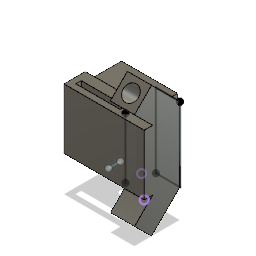
batt basee v1 (Autodesk Fusion 360 design; units mm, degrees)
Autodesk Fusion 360 part; units mm, degrees
sketch "Sketch1" plane through (0, 0, 0) normal (0, 0, 1) x (1, 0, 0)
  line L0 (0, 0) -> (13.5, 0)
  line L1 (13.5, 0) -> (13.5, 13.5)
  line L2 (13.5, 13.5) -> (0, 13.5)
  line L3 (0, 13.5) -> (0, 0)
  line L4 (-3.75, -3.75) -> (17.25, -3.75)
  line L5 (17.25, -3.75) -> (17.25, 17.25)
  line L6 (17.25, 17.25) -> (-3.75, 17.25)
  line L7 (-3.75, 17.25) -> (-3.75, -3.75)
  dimension "d1" = 13.5
  dimension "d2" = 13.5
  dimension "d3" = 3.75
  constraint horizontal L0
  constraint vertical L1
  constraint horizontal L2
  constraint vertical L3
  constraint coincident L0.start L3.end
  measures "d1" distance of L0.start L2.end
  measures "d2" distance of L1.end L2.end
  measures "d43" distance of L0.start
  measures "d47" distance of L0.start
extrude "Extrude1" add sketch "Sketch1" along normal blind 20
sketch "Sketch2" plane through (0, 0, 20) normal (0, 0, 1) x (1, 0, 0)
  line L0 (0, 0) -> (0, 13.5)
  line L1 (0, 13.5) -> (13.5, 13.5)
  line L2 (13.5, 13.5) -> (13.5, 0)
  line L3 (13.5, 0) -> (0, 0)
  line L4 (-3.75, 17.25) -> (-3.75, -3.75)
  line L5 (-3.75, -3.75) -> (17.25, -3.75)
  line L6 (17.25, -3.75) -> (17.25, 17.25)
  line L7 (17.25, 17.25) -> (-3.75, 17.25)
  line L8 (6.75, 6.75) -> (6.75, 21.75)
  line L9 (6.75, 6.75) -> (6.75, -8.25)
  line L10 (6.75, 6.75) -> (17.25, 6.75)
  line L11 (17.25, 6.75) -> (17.25, 21.75)
  line L12 (17.25, 21.75) -> (6.75, 21.75)
  line L13 (6.75, -8.25) -> (17.25, -8.25)
  line L14 (17.25, -8.25) -> (17.25, 6.75)
  line L15 (6.75, 6.75) -> (-3.75, 6.75)
  line L16 (-3.75, 6.75) -> (-3.75, 21.75)
  line L17 (-3.75, 21.75) -> (6.75, 21.75)
  line L18 (6.75, -8.25) -> (-3.75, -8.25)
  line L19 (-3.75, -8.25) -> (-3.75, 6.75)
  dimension "d6" = 15
  dimension "d7" = 15
  dimension "d8" = 15
  constraint perpendicular L1 L8
  constraint perpendicular L5 L9
  constraint midpoint L6 L10.end
  constraint perpendicular L6 L10
  constraint perpendicular L10 L11
  constraint perpendicular L8 L12
  constraint perpendicular L9 L13
  constraint perpendicular L10 L14
  constraint midpoint L4 L15.end
  constraint perpendicular L7 L16
  constraint perpendicular L9 L18
  constraint perpendicular L15 L19
  measures "d6" distance of L8.start L8.end
  measures "d7" distance of L8.start L9.end
  measures "d8" distance of L15.end L16.end
extrude "Extrude2" add sketch "Sketch2" along normal blind 3
sketch "Sketch3" plane through (17.25, 0, 0) normal (1, 0, 0) x (0, 0, -1)
  line L0 (0, -3.75) -> (0, 17.25)
  line L1 (0, 17.25) -> (-20, 17.25)
  line L2 (-20, 17.25) -> (-20, 21.75)
  line L3 (-20, 21.75) -> (-23, 21.75)
  line L4 (-23, 21.75) -> (-23, -8.25)
  line L5 (-23, -8.25) -> (-20, -8.25)
  line L6 (-20, -8.25) -> (-20, -3.75)
  line L7 (-20, -3.75) -> (0, -3.75)
  line L8 (-23, 6.75) -> (0, 6.75)
  line L9 (-3, 6.75) -> (-13.6066, -3.8566)
  line L10 (-7.2426, 10.9926) -> (-17.8492, 0.386)
  line L11 (1.2426, 2.5074) -> (-9.364, -8.0992)
  line L12 (-7.2426, 2.5074) -> (-17.8492, 13.114)
  line L13 (-3, 6.75) -> (-13.6066, 17.3566)
  line L14 (1.2426, 10.9926) -> (-9.364, 21.5992)
  line L15 (-3, 6.75) -> (1.2426, 10.9926)
  line L16 (-3, 6.75) -> (1.2426, 2.5074)
  line L17 (-17.8492, 13.114) -> (-9.364, 21.5992)
  line L18 (-17.8492, 0.386) -> (-9.364, -8.0992)
  dimension "d14" = 45
  dimension "d15" = 6
  dimension "d16" = -6
  dimension "d17" = 15
  dimension "d18" = 20
  constraint midpoint L4 L8.start
  constraint midpoint L0 L8.end
  constraint symmetric L8 L9.start L13.start
  constraint symmetric L8 L9.end L13.end
  constraint symmetric L8 L10.start L12.start
  constraint symmetric L8 L10.end L12.end
  constraint symmetric L8 L11.start L14.start
  constraint symmetric L8 L11.end L14.end
  constraint perpendicular L14 L15
  constraint perpendicular L14 L17
  measures "d14" angle of L8 L9
  measures "d17" distance of L9.start L9.end
  measures "d18" distance of L8.start L9.start
extrude "Extrude3" add sketch "Sketch3" along normal blind 12 contours L0 L7 L9 L11 L16 | L7 L9 L11 L18 | L7 L9 L18 | L7 L9 L10 L12 L18 | L8 L9 L12 | L8 L10 L13 | L0 L1 L13 L14 L15 | L1 L10 L12 L13 L17 | L1 L13 L14 L17 | L1 L13 L17
sketch "Sketch4" plane through (0, -8.7316, 8.7316) normal (0, -0.707107, 0.707107) x (1, 0, 0)
  line L0 (17.25, 12.8943) -> (17.25, 7.045)
  line L1 (17.25, 7.045) -> (17.25, 0.8943)
  line L2 (17.25, 0.8943) -> (29.25, 0.8943)
  line L3 (29.25, 0.8943) -> (29.25, 12.8943)
  line L4 (29.25, 12.8943) -> (17.25, 12.8943)
  circle A0 centre (23.25, 6.8943) radius 3.8
  dimension "d21" = 7.6
  measures "d21" diameter of A0
extrude "Extrude4" cut sketch "Sketch4" against normal blind 10 contours A0
sketch "Sketch5" plane through (0, 15.4816, 15.4816) normal (0, 0.707107, 0.707107) x (1, 0, 0)
  line L0 (17.25, 2.5009) -> (17.25, -3.3483)
  line L1 (17.25, -3.3483) -> (29.25, -3.3483)
  line L2 (29.25, -3.3483) -> (29.25, 8.6517)
  line L3 (29.25, 8.6517) -> (17.25, 8.6517)
  line L4 (17.25, 8.6517) -> (17.25, 2.5009)
  circle A0 centre (23.25, 2.6517) radius 3.8
  dimension "d24" = 7.6
  measures "d24" diameter of A0
extrude "Extrude5" cut sketch "Sketch5" against normal blind 10 contours A0
extrude "Extrude6" add 1 faces at (18.1088, -5.6239, 11.8393) along direction (0, -0.707107, 0.707107) blind 25
extrude "Extrude7" add 1 faces at (18.1088, 19.1239, 11.8393) along direction (0, 0.707107, 0.707107) blind 25
extrude "Extrude8" add 1 faces at (17.25, 6.75, 19.1618) along direction (1, 0, 0) blind 12
sketch "Sketch6" plane through (0, 0, 23) normal (0, 0, 1) x (1, 0, 0)
  line L0 (-3.75, -8.25) -> (17.25, -8.25)
  line L1 (17.25, -8.25) -> (17.25, -4.7647)
  line L2 (17.25, -4.7647) -> (29.25, -4.7647)
  line L3 (29.25, -4.7647) -> (29.25, 18.2647)
  line L4 (29.25, 18.2647) -> (17.25, 18.2647)
  line L5 (17.25, 18.2647) -> (17.25, 21.75)
  line L6 (17.25, 21.75) -> (-3.75, 21.75)
  line L7 (-3.75, 21.75) -> (-3.75, -8.25)
  line L8 (17.25, -8.25) -> (-3.75, -8.25)
  line L9 (-3.75, -8.25) -> (-3.75, 21.75)
  line L10 (-3.75, 21.75) -> (17.25, 21.75)
  line L11 (17.25, 21.75) -> (17.25, -8.25)
  constraint horizontal L8
  constraint vertical L9
  constraint horizontal L10
  constraint vertical L11
  constraint coincident L6.end L7.start
  constraint coincident L0.end L1.start
extrude "Extrude9" add sketch "Sketch6" along normal blind 5 contours L0 L1 L5 L6 L7 L8 L9 L10 L11
sketch "Sketch7" plane through (17.25, 0, 0) normal (1, 0, 0) x (0, 0, -1)
  line L0 (-26.4853, -8.25) -> (-23, -4.7647)
  line L1 (-23, -4.7647) -> (-23, 18.2647)
  line L2 (-23, 18.2647) -> (-26.4853, 21.75)
  line L3 (-26.4853, 21.75) -> (-28, 21.75)
  line L4 (-28, 21.75) -> (-28, -8.25)
  line L5 (-28, -8.25) -> (-26.4853, -8.25)
  line L6 (-28, -8.25) -> (-28, 21.75)
  constraint coincident L4.end L5.start
  constraint coincident L3.end L4.start
sketch "Sketch8" plane through (29.25, 0, 0) normal (1, 0, 0) x (0, 0, -1)
  line L0 (-23, -4.7647) -> (-35.5269, -17.2916)
  line L1 (-35.5269, -17.2916) -> (-27.0416, -25.7769)
  line L2 (-27.0416, -25.7769) -> (0, 1.2647)
  line L3 (0, 1.2647) -> (0, 3.75)
  line L4 (0, 3.75) -> (-3, 6.75)
  line L5 (-3, 6.75) -> (0, 9.75)
  line L6 (0, 9.75) -> (0, 12.2353)
  line L7 (0, 12.2353) -> (-27.0416, 39.2769)
  line L8 (-27.0416, 39.2769) -> (-35.5269, 30.7916)
  line L9 (-35.5269, 30.7916) -> (-23, 18.2647)
  line L10 (-23, 18.2647) -> (-23, -4.7647)
  line L11 (-29.2635, 24.5282) -> (-29.2635, -11.0282)
  line L12 (-29.2635, 24.5282) -> (-29.9706, 25.2353)
  line L13 (-29.2635, -11.0282) -> (-29.9706, -11.7353)
  line L14 (-29.9706, -11.7353) -> (-29.9706, 25.2353)
  line L15 (-29.9706, 25.2353) -> (-30.6777, 25.9424)
  line L16 (-29.9706, -11.7353) -> (-30.6777, -12.4424)
  line L17 (-30.6777, -12.4424) -> (-30.6777, 25.9424)
  dimension "d35" = 1
  dimension "d36" = 1
  dimension "d37" = 1
  dimension "d38" = 1
  constraint midpoint L9 L11.start
  constraint midpoint L0 L11.end
  constraint parallel L9 L12
  constraint parallel L0 L13
  constraint parallel L9 L15
  constraint parallel L0 L16
  measures "d35" distance of L11.start L12.end
  measures "d36" distance of L11.end L13.end
  measures "d37" distance of L12.end L15.end
  measures "d38" distance of L13.end L16.end
extrude "Extrude10" add sketch "Sketch8" against normal blind 33 contours L0 L9 L10 L11 | L0 L9 L11 L12 L13 L14 | L0 L9 L14 L15 L16 L17
sketch "Sketch9" plane through (-3.75, 0, 0) normal (-1, 0, 0) x (0, 0, 1)
  line L0 (26.4853, 21.75) -> (20, 21.75)
  line L1 (20, 21.75) -> (20, 17.25)
  line L2 (20, 17.25) -> (0, 17.25)
  line L3 (0, 17.25) -> (0, -3.75)
  line L4 (0, -3.75) -> (20, -3.75)
  line L5 (20, -3.75) -> (20, -8.25)
  line L6 (20, -8.25) -> (26.4853, -8.25)
  line L7 (26.4853, -8.25) -> (30.6777, -12.4424)
  line L8 (30.6777, -12.4424) -> (30.6777, 25.9424)
  line L9 (30.6777, 25.9424) -> (26.4853, 21.75)
  line L10 (26.4853, 21.75) -> (35, 21.75)
  line L11 (26.4853, -8.25) -> (40, -8.25)
  constraint coincident L0.start L9.end
  constraint perpendicular L8 L10
  constraint coincident L6.end L7.start
  constraint perpendicular L8 L11
extrude "Extrude11" cut sketch "Sketch9" against normal blind 40 contours L8 L9 L10 | L7 L8 L11
sketch "Sketch10" plane through (29.25, 0, 0) normal (1, 0, 0) x (0, 0, -1)
  line L0 (-30.6777, -8.25) -> (-26.4853, -8.25)
  line L1 (-26.4853, -8.25) -> (-35.5269, -17.2916)
  line L2 (-35.5269, -17.2916) -> (-27.0416, -25.7769)
  line L3 (-27.0416, -25.7769) -> (0, 1.2647)
  line L4 (0, 1.2647) -> (0, 3.75)
  line L5 (0, 3.75) -> (-3, 6.75)
  line L6 (-3, 6.75) -> (0, 9.75)
  line L7 (0, 9.75) -> (0, 12.2353)
  line L8 (0, 12.2353) -> (-27.0416, 39.2769)
  line L9 (-27.0416, 39.2769) -> (-35.5269, 30.7916)
  line L10 (-35.5269, 30.7916) -> (-26.4853, 21.75)
  line L11 (-26.4853, 21.75) -> (-30.6777, 21.75)
  line L12 (-30.6777, 21.75) -> (-30.6777, -8.25)
  line L13 (-31.2843, -21.5343) -> (-17.1421, -7.3921)
  line L14 (-17.1421, -7.3921) -> (-12.8995, -11.6348)
  line L15 (-35.5269, -17.2916) -> (-21.3848, -3.1495)
  line L16 (-21.3848, -3.1495) -> (-17.1421, -7.3921)
  line L17 (-12.8995, -11.6348) -> (-12.8995, 25.1348)
  line L18 (-30.6777, 6.75) -> (-12.8995, 6.75)
  line L19 (-31.2843, 35.0343) -> (-17.1421, 20.8921)
  line L20 (-35.5269, 30.7916) -> (-21.3848, 16.6495)
  line L21 (-21.3848, 16.6495) -> (-17.1421, 20.8921)
  line L22 (-27.0416, 39.2769) -> (0, 12.2353)
  line L23 (-17.1421, 20.8921) -> (-12.8995, 25.1348)
  line L24 (-35.5269, 30.7916) -> (-27.0416, 39.2769)
  dimension "d43" = 20
  dimension "d44" = 20
  constraint midpoint L2 L13.start
  constraint perpendicular L2 L13
  constraint coincident L3 L14.end
  constraint perpendicular L3 L14
  constraint coincident L1.end L2.start
  constraint perpendicular L2 L15
  constraint coincident L8 L17.end
  constraint vertical L17
  constraint midpoint L12 L18.start
  constraint midpoint L17 L18.end
  constraint symmetric L1.end L18 L9.end
  constraint symmetric L2.end L18 L8.end
  constraint symmetric L3.end L18 L7.end
  constraint symmetric L13.start L18 L19.start
  constraint symmetric L13.end L18 L19.end
  constraint symmetric L14.end L18 L17.end
  constraint symmetric L15.end L18 L20.end
  measures "d43" distance of L13.start L13.end
  measures "d44" distance of L1.end L15.end
extrude "Extrude12" cut sketch "Sketch10" against normal blind 12 contours L3 L4 L5 L6 L7 L8 L17 L22
sketch "Sketch11" plane through (0, 0, 12.8995) normal (0, 0, -1) x (-1, 0, 0)
  ellipse E0 centre (-23.25, 16.6495) end of major axis (-23.25, 11.2755) minor radius 3.8
  ellipse E1 centre (-23.25, -3.1495) end of major axis (-23.25, -8.5235) minor radius 3.8
  line L0 (-29.25, 25.1348) -> (-29.25, -11.6348)
  line L1 (-29.25, -11.6348) -> (-17.25, -11.6348)
  line L2 (-17.25, -11.6348) -> (-17.25, -3.75)
  line L3 (-17.25, -3.75) -> (-17.25, 17.25)
  line L4 (-17.25, 17.25) -> (-17.25, 25.1348)
  line L5 (-17.25, 25.1348) -> (-29.25, 25.1348)
  line L6 (-17.25, -11.6348) -> (-29.25, -11.6348)
  line L7 (-29.25, -11.6348) -> (-29.25, 25.1348)
  line L8 (-29.25, 25.1348) -> (-17.25, 25.1348)
  line L9 (-17.25, 25.1348) -> (-17.25, -11.6348)
  constraint horizontal L6
  constraint vertical L7
  constraint horizontal L8
  constraint vertical L9
  constraint coincident L0.start L5.end
  constraint coincident L1.end L2.start
sketch "Sketch12" plane through (29.25, 0, 0) normal (1, 0, 0) x (0, 0, -1)
  line L0 (-12.8995, -11.6348) -> (-12.8995, 25.1348)
  line L1 (-12.8995, 25.1348) -> (-27.0416, 39.2769)
  line L2 (-27.0416, 39.2769) -> (-35.5269, 30.7916)
  line L3 (-35.5269, 30.7916) -> (-26.4853, 21.75)
  line L4 (-26.4853, 21.75) -> (-30.6777, 21.75)
  line L5 (-30.6777, 21.75) -> (-30.6777, -8.25)
  line L6 (-30.6777, -8.25) -> (-26.4853, -8.25)
  line L7 (-26.4853, -8.25) -> (-35.5269, -17.2916)
  line L8 (-35.5269, -17.2916) -> (-27.0416, -25.7769)
  line L9 (-27.0416, -25.7769) -> (-12.8995, -11.6348)
  line L10 (-31.2843, -21.5343) -> (-18.5563, -8.8063)
  line L11 (-18.5563, -8.8063) -> (-14.3137, -13.049)
  line L12 (-18.5563, -8.8063) -> (-30.6777, 3.315)
  line L13 (-30.6777, 6.75) -> (-12.8995, 6.75)
  line L14 (-18.5563, 22.3063) -> (-30.6777, 10.185)
  line L15 (-18.5563, 22.3063) -> (-14.3137, 26.549)
  dimension "d47" = 18
  constraint midpoint L8 L10.start
  constraint perpendicular L8 L10
  constraint coincident L9 L11.end
  constraint perpendicular L9 L11
  constraint coincident L5 L12.end
  constraint perpendicular L10 L12
  constraint midpoint L5 L13.start
  constraint midpoint L0 L13.end
  constraint symmetric L10.end L13 L14.start
  constraint symmetric L11.end L13 L15.end
  constraint symmetric L12.end L13 L14.end
  measures "d47" distance of L10.start L10.end
extrude "Extrude13" add sketch "Sketch12" against normal blind 12 contours L0 L5 L9 L11 L12 L13 | L0 L1 L5 L13 L14 L15
extrude "Extrude14" cut 1 faces at (4.5, 9, 20) along direction (0, 0, 1) blind 5
sketch "Sketch13" plane through (0, -8.25, 0) normal (0, -1, 0) x (1, 0, 0)
  line L0 (17.25, 20) -> (17.25, 26.4853)
  line L1 (17.25, 26.4853) -> (29.25, 26.4853)
  line L2 (29.25, 26.4853) -> (29.25, 30.6777)
  line L3 (6.75, 20) -> (6.75, 24.9777)
  line L4 (6.75, 24.9777) -> (6.75, 25.9777)
extrude "Extrude15" add 1 faces at (-3.75, 10.25, 6.6667) along direction (-1, 0, 0) blind 9
extrude "Extrude16" cut 1 faces at (0, 9, 8.3333) along direction (-1, 0, 0) blind 9
extrude "Extrude17" add 1 faces at (13.5, 4.5, 8.3333) along direction (-1, 0, 0) blind 9
extrude "Extrude18" cut 1 faces at (4.5, 4.5, 8.3333) along direction (1, 0, 0) blind 8.25
extrude "Extrude19" add 1 faces at (-9, 9, 8.3333) along direction (1, 0, 0) blind 8.25
extrude "Extrude20" add 1 faces at (3.75, 9, 25) along direction (0, 0, -1) blind 25
sketch "Sketch14" plane through (0, 0, 0) normal (0, 0, -1) x (-1, 0, 0)
  line L0 (-17.25, 17.25) -> (-17.25, -3.75)
  line L1 (-17.25, -3.75) -> (12.75, -3.75)
  line L2 (12.75, -3.75) -> (12.75, 17.25)
  line L3 (12.75, 17.25) -> (-17.25, 17.25)
  line L4 (-9, 13.5) -> (4.5, 13.5)
  line L5 (4.5, 13.5) -> (4.5, 0)
  line L6 (4.5, 0) -> (-9, 0)
  line L7 (-9, 0) -> (-9, 13.5)
  line L8 (-17.25, 25.1348) -> (-17.25, -11.6348)
  dimension "d70" = 13.5
  dimension "d71" = 13.5
  dimension "d72" = 8.25
  dimension "d73" = 8.25
  dimension "d74" = 3.75
  dimension "d75" = 21
  dimension "d76" = 13.5
  dimension "d77" = 3.75
  constraint horizontal L4
  constraint vertical L5
  constraint horizontal L6
  constraint vertical L7
  measures "d70" distance of L4.start L6.end
  measures "d71" distance of L4.start L4.end
  measures "d72" distance of L2 L5
  measures "d73" distance of L7 L8
  measures "d74" distance of L3 L4
  measures "d75" distance of L1.end L2.end
  measures "d76" distance of L5.end L6.end
  measures "d77" distance of L1 L6
extrude "Extrude21" cut sketch "Sketch14" against normal blind 20 contours L4 L5 L6 L7
sketch "Sketch15" plane through (0, -8.25, 0) normal (0, -1, 0) x (1, 0, 0)
  line L0 (-12.75, 20) -> (17.25, 20)
  line L1 (17.25, 20) -> (17.25, 26.4853)
  line L2 (17.25, 26.4853) -> (29.25, 26.4853)
  line L3 (29.25, 26.4853) -> (29.25, 30.6777)
  line L4 (29.25, 30.6777) -> (-12.75, 30.6777)
  line L5 (-12.75, 30.6777) -> (-12.75, 20)
  line L6 (-12.75, 20) -> (17.25, 20)
  line L7 (2.25, 20) -> (2.25, 30.6777)
  line L8 (2.25, 30.6777) -> (2.25, 27.6777)
  line L9 (2.25, 27.6777) -> (13.25, 27.6777)
  line L10 (2.25, 27.6777) -> (-8.75, 27.6777)
  line L11 (-8.75, 27.6777) -> (-8.75, 24.9777)
  line L12 (-8.75, 24.9777) -> (13.25, 24.9777)
  line L13 (13.25, 24.9777) -> (13.25, 27.6777)
  line L14 (2.25, 24.9777) -> (2.25, 21.9777)
  line L15 (2.25, 20) -> (2.25, 21.9777)
  dimension "d80" = 3
  dimension "d81" = 11
  dimension "d82" = 11
  dimension "d83" = 2.7
  dimension "d84" = 22
  dimension "d85" = 3
  dimension "d86" = 1.9777
  constraint coincident L0.start L5.end
  constraint coincident L0.end L1.start
  constraint midpoint L0 L7.start
  constraint coincident L4 L7.end
  constraint perpendicular L4 L7
  constraint perpendicular L4 L8
  constraint perpendicular L7 L9
  constraint perpendicular L8 L10
  constraint perpendicular L10 L11
  constraint perpendicular L11 L12
  constraint midpoint L12 L14.start
  constraint perpendicular L12 L14
  measures "d80" distance of L7.end L8.end
  measures "d81" distance of L8.end L9.end
  measures "d82" distance of L8.end L10.end
  measures "d83" distance of L10.end L11.end
  measures "d84" distance of L11.end L12.end
  measures "d85" distance of L14.start L14.end
  measures "d86" distance of L7.start L14.end
extrude "Extrude22" cut sketch "Sketch15" against normal blind 36 contours L7 L10 L11 L12 | L7 L9 L12 L13
extrude "Extrude23" cut 1 faces at (4.5, 4.5, 20) along direction (0, 0, 1) blind 1.978
extrude "Extrude24" cut 1 faces at (-10, 9, 0) along direction (0, 0, 1) blind 1.978
extrude "Extrude25" cut 1 faces at (13.25, 1.75, 25.8777) along direction (1, 0, 0) blind 1
extrude "Extrude26" add 1 faces at (-8.75, 1.75, 26.7777) along direction (1, 0, 0) blind 1
extrude "Extrude27" cut 1 faces at (9, 4.5, 8.6447) along direction (1, 0, 0) blind 1
extrude "Extrude28" add 1 faces at (-4.5, 9, 8.6447) along direction (1, 0, 0) blind 1
extrude "Extrude29" cut 1 faces at (-12.75, 10.25, 7.9853) along direction (1, 0, 0) blind 2
sketch "Sketch16" plane through (0, -3.75, 0) normal (0, -1, 0) x (1, 0, 0)
  line L0 (-10.75, 20) -> (-10.75, 1.978)
  line L1 (-10.75, 1.978) -> (17.25, 1.978)
  line L2 (17.25, 1.978) -> (17.25, 12.8995)
  line L3 (17.25, 12.8995) -> (17.25, 20)
  line L4 (17.25, 20) -> (-10.75, 20)
  line L5 (3.25, 1.978) -> (3.25, 8.6447)
  circle A0 centre (3.25, 8.6447) radius 1.45
  circle A1 centre (3.25, 15.3113) radius 1.45
  dimension "d103" = 6.6667
  dimension "d104" = 2.9
  dimension "d105" = 2.9
  dimension "d106" = 6.6667
  constraint midpoint L1 L5.start
  constraint perpendicular L1 L5
  constraint coincident L5.end A0.centre
  measures "d103" distance of L5.start L5.end
  measures "d104" diameter of A0
  measures "d105" diameter of A1
  measures "d106" distance of L5.end A1.centre
extrude "Extrude30" cut sketch "Sketch16" against normal blind 31 contours A0 | A1
equation "d103 = ( 20 / 3 ) * 1 mm"
equation "d106 = ( 20 / 3 ) * 1 mm"
